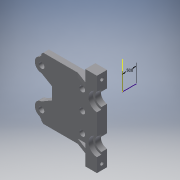
# Autodesk Inventor part: Hotend mount
Saved by Autodesk Inventor 2016 (Build 200138000, 138)
## iProperties
Created: 2016-06-02
Part Number: Hotend mount
Material: Generic
Document SubType Name: Modeling
Designer: Scott
Density: 1 g/cm^3
Appearance: Default
Author: Scott
Autodesk Inventor part; units mm, degrees
ref_plane "YZ Plane" through (0, 0, 0) normal (1, 0, 0) x (0, 1, 0)
ref_plane "XZ Plane" through (0, 0, 0) normal (0, 1, 0) x (-1, 0, 0)
sketch "Sketch1" plane through (0, 0, 0) normal (0, 0, 1) x (1, 0, 0)
  line L0 (-13.6843, -5.4848) -> (-23.1843, -10.9697) projected
  line L1 (-23.1843, -10.9697) -> (-32.6843, -5.4848) projected
  line L2 (-32.6843, -5.4848) -> (-32.6843, 5.4848) projected
  line L3 (-32.6843, 5.4848) -> (-23.1843, 10.9697) projected
  line L4 (-23.1843, 10.9697) -> (-13.6843, 5.4848) projected
  line L5 (-13.6843, 5.4848) -> (-13.6843, -5.4848) projected
  circle A0 centre (13.3507, 17.0193) radius 2.54 projected
  circle A1 centre (13.3507, -17.4028) radius 2.54 projected
  circle A2 centre (13.3507, 0) radius 2.54 projected
  circle A3 centre (-23.0489, 17.0193) radius 2.54 projected
  circle A4 centre (-23.2, -17.4028) radius 2.54 projected
  line L6 (-54.6393, -27.54) -> (18.4307, -27.54) projected
  line L7 (18.4307, -27.54) -> (18.4307, 27.54) projected
  line L8 (-54.6393, 27.54) -> (18.4307, 27.54) projected
  line L9 (-54.6393, -27.54) -> (-54.6393, 27.54) projected
  arc A5 (-23.1843, 23.0689) -> (-23.1843, 10.9697) centre (-23.0489, 17.0193) ccw
  line L10 (-23.1843, 10.9697) -> (-13.6843, 5.4848)
  line L11 (-13.6843, 5.4848) -> (-13.6843, -5.4848)
  line L12 (-13.6843, -5.4848) -> (-23.1843, -10.9697)
  line L13 (-23.1843, -23.6032) -> (-23.1843, -27.54)
  line L14 (-23.1843, 23.0689) -> (-23.1843, 27.54)
  line L15 (-23.1843, -27.54) -> (18.4307, -27.54)
  line L16 (18.4307, -27.54) -> (18.4307, 27.54)
  line L17 (18.4307, 27.54) -> (-23.1843, 27.54)
  arc A6 (-23.1843, -10.9697) -> (-23.1843, -23.6032) centre (-22.7708, -17.2864) ccw
  point P0 (0, 0)
  constraints: 16 end point, 5 collinear, 4 point on circle, 4 point on line, 2 centre point, 1 coincident, 1 horizontal, 1 perpendicular
extrude "Extrusion1" add sketch "Sketch1" along normal blind 5.08 contours L5 L4 A5 L14 L8 L7 L6 L13 A6 L0
chamfer "Chamfer1" distance 1.5875 angle 45 4 edges at (-23.1843, -27.54, 2.54) (-23.1843, 27.54, 2.54) (-23.1843, 23.0689, 2.54) (-23.1843, -23.6032, 2.54)
sketch "Sketch2" plane through (18.4307, -27.54, 0) normal (1, 0, 0) x (0, 0, -1)
  line L0 (25.4, 55.08) -> (25.4, 29.5535) projected
  line L1 (25.4, 29.5535) -> (38.1, 29.5535)
  point P0 (0, 27.54)
  dimension "d5" = 12.7
  constraints: 2 end point, 1 horizontal
  measures "d5" distance of L0.end L1.end
sketch "Sketch3" plane through (0, 0, 5.08) normal (0, 0, 1) x (1, 0, 0)
  line L0 (-23.1843, 25.9525) -> (-21.5968, 27.54) projected
  line L1 (-23.1843, 25.9525) -> (-23.1843, 24.6564) projected
  line L2 (-24.753, 22.8255) -> (-23.1843, 24.6564) projected
  arc A0 (-24.753, 22.8255) -> (-23.1843, 10.9697) centre (-23.0489, 17.0193) ccw projected
  line L3 (-23.1843, 10.9697) -> (-13.6843, 5.4848) projected
  line L4 (-13.6843, 5.4848) -> (-13.6843, -5.4848) projected
  line L5 (-13.6843, -5.4848) -> (-23.1843, -10.9697) projected
  arc A1 (-23.1843, -10.9697) -> (-24.7429, -23.3017) centre (-22.7708, -17.2864) ccw projected
  line L6 (-23.1843, -25.1907) -> (-24.7429, -23.3017) projected
  line L7 (-23.1843, -25.1907) -> (-23.1843, -25.9525) projected
  line L8 (-21.5968, -27.54) -> (-23.1843, -25.9525) projected
  line L9 (-21.5968, -27.54) -> (18.4307, -27.54) projected
  line L10 (18.4307, -27.54) -> (18.4307, 27.54) projected
  line L11 (18.4307, 27.54) -> (-21.5968, 27.54) projected
  circle A2 centre (-23.2, -17.4028) radius 2.54 projected
  circle A3 centre (-23.0489, 17.0193) radius 2.54 projected
  circle A4 centre (13.3507, 0) radius 2.54 projected
  circle A5 centre (13.3507, -17.4028) radius 2.54 projected
  circle A6 centre (13.3507, 17.0193) radius 2.54 projected
  line L12 (18.4307, -17.4028) -> (24.9307, -17.4028)
  line L13 (24.9307, -17.4028) -> (30.9307, -17.4028)
  arc A7 (30.9307, -11.4028) -> (30.9307, -23.4028) centre (30.9307, -17.4028) ccw
  line L14 (30.9307, -23.4028) -> (30.9307, -27.54)
  line L15 (30.9307, -27.54) -> (18.4307, -27.54)
  line L16 (18.4307, 0) -> (20.9229, 0)
  line L17 (18.4307, 17.4028) -> (24.9307, 17.4028)
  line L18 (24.9307, 17.4028) -> (30.9307, 17.4028)
  arc A8 (30.9307, 23.4028) -> (30.9307, 11.4028) centre (30.9307, 17.4028) ccw
  line L19 (30.9307, 23.4028) -> (30.9307, 27.54)
  line L20 (30.9307, 27.54) -> (18.4307, 27.54)
  line L21 (30.9307, -11.4028) -> (30.9307, 11.4028)
  point P0 (0, 0)
  dimension "d6" = 6.5
  dimension "d7" = 6
  dimension "d8" = 6
  constraints: 20 end point, 7 symmetric about line, 5 point on circle, 3 point on line, 2 centre point, 2 coincident, 2 perpendicular, 2 vertical, 1 horizontal, 1 midpoint, 1 other
  measures "d6" distance of L12.start L12.end
  measures "d7" distance of L12.end L13.end
  measures "d8" radius of A7
ref_plane "Work Plane1" through (-54.6393, -27.54, 0) normal (0, 0, 1) x (1, 0, 0)
extrude "Extrusion2" add sketch "Sketch3" against normal up to surface (5.08 mm away) contours L20 L19 A8 L17 L10 | L17 A8 L21 A7 L12 L10 | L12 A7 L14 L15 L10
sketch "Sketch4" plane through (0, 0, 5.08) normal (0, 0, 1) x (1, 0, 0)
  line L0 (-23.1843, 25.9525) -> (-21.5968, 27.54) projected
  line L1 (-23.1843, 25.9525) -> (-23.1843, 24.6564) projected
  line L2 (-24.753, 22.8255) -> (-23.1843, 24.6564) projected
  arc A0 (-24.753, 22.8255) -> (-23.1843, 10.9697) centre (-23.0489, 17.0193) ccw projected
  line L3 (-23.1843, 10.9697) -> (-13.6843, 5.4848) projected
  line L4 (-13.6843, 5.4848) -> (-13.6843, -5.4848) projected
  line L5 (-13.6843, -5.4848) -> (-23.1843, -10.9697) projected
  arc A1 (-23.1843, -10.9697) -> (-24.7429, -23.3017) centre (-22.7708, -17.2864) ccw projected
  line L6 (-23.1843, -25.1907) -> (-24.7429, -23.3017) projected
  line L7 (-23.1843, -25.1907) -> (-23.1843, -25.9525) projected
  line L8 (-21.5968, -27.54) -> (-23.1843, -25.9525) projected
  line L9 (-21.5968, -27.54) -> (30.9307, -27.54) projected
  line L10 (30.9307, -27.54) -> (30.9307, -23.4028) projected
  arc A2 (30.9307, -11.4028) -> (30.9307, -23.4028) centre (30.9307, -17.4028) ccw projected
  line L11 (30.9307, -11.4028) -> (30.9307, 11.4028) projected
  arc A3 (30.9307, 23.4028) -> (30.9307, 11.4028) centre (30.9307, 17.4028) ccw projected
  line L12 (30.9307, 23.4028) -> (30.9307, 27.54) projected
  line L13 (30.9307, 27.54) -> (-21.5968, 27.54) projected
  circle A4 centre (-23.2, -17.4028) radius 2.54 projected
  circle A5 centre (-23.0489, 17.0193) radius 2.54 projected
  circle A6 centre (13.3507, 0) radius 2.54 projected
  circle A7 centre (13.3507, -17.4028) radius 2.54 projected
  circle A8 centre (13.3507, 17.0193) radius 2.54 projected
  line L14 (30.9307, -23.4028) -> (30.9307, -27.54) projected
  arc A9 (30.9307, -9.4028) -> (30.9307, -25.4028) centre (30.9307, -17.4028) ccw
  arc A10 (30.9307, 23.4028) -> (30.9307, 11.4028) centre (30.9307, 17.4028) ccw projected
  line L15 (30.9307, -11.4028) -> (30.9307, 11.4028) projected
  arc A11 (30.9307, 25.4028) -> (30.9307, 9.4028) centre (30.9307, 17.4028) ccw
  line L16 (-21.5968, -27.54) -> (30.9307, -27.54) projected
  line L17 (20.0107, -27.54) -> (20.0107, 27.54)
  line L18 (30.9307, 27.54) -> (-21.5968, 27.54) projected
  line L19 (20.0107, -26.7462) -> (20.0107, -27.54)
  line L20 (-21.5968, -27.54) -> (30.9307, -27.54) projected
  line L21 (20.0107, -27.54) -> (30.9307, -27.54)
  line L22 (30.9307, -27.54) -> (30.9307, -23.4028) projected
  line L23 (30.9307, -25.4028) -> (30.9307, -27.54)
  line L24 (30.9307, -9.4028) -> (30.9307, 9.4028)
  line L25 (20.0107, 27.54) -> (30.9307, 27.54)
  line L26 (30.9307, 27.54) -> (30.9307, 25.4028)
  line L27 (30.9307, 23.4028) -> (30.9307, 27.54) projected
  point P0 (0, 0)
  dimension "d11" = 8
  dimension "d12" = 8
  constraints: 14 end point, 5 point on line, 4 collinear, 4 point on circle, 2 centre point, 2 coincident, 2 perpendicular, 1 vertical
  measures "d11" radius of A9
  measures "d12" radius of A11
extrude "Extrusion3" add sketch "Sketch4" along normal blind 4 contours L13 L12 A11 L11 A9 L10 L9 L17
sketch "Sketch5" plane through (-21.5968, -27.54, 0) normal (0, -1, 0) x (1, 0, 0)
  point P0 (21.5968, 0)
sketch "Sketch6" plane through (-21.5968, -27.54, 0) normal (0, -1, 0) x (1, 0, 0)
  line L0 (0, 0) -> (0, 5.08) projected
  line L1 (0, 0) -> (52.5275, 0) projected
  line L2 (52.5275, 0) -> (52.5275, 9.08) projected
  line L3 (41.6075, 9.08) -> (52.5275, 9.08) projected
  line L4 (41.6075, 5.08) -> (41.6075, 9.08) projected
  line L5 (0, 5.08) -> (41.6075, 5.08) projected
  line L6 (41.6075, 5.08) -> (41.6075, 9.08) projected
  line L7 (41.6075, 9.08) -> (30.9206, 5.08)
  line L8 (0, 5.08) -> (41.6075, 5.08) projected
  point P0 (21.5968, 0)
  constraints: 2 end point, 1 point on line
extrude "Extrusion4" add sketch "Sketch6" against normal blind 4 contours L7 L4 L5
sketch "Sketch7" plane through (-21.5968, 27.54, 5.08) normal (0, 1, 0) x (1, 0, 0)
  line L0 (41.6075, 0) -> (41.6075, -4) projected
  line L1 (30.9206, 0) -> (41.6075, 0) projected
  line L2 (30.9206, 0) -> (41.6075, -4) projected
  point P0 (21.5968, 5.08)
extrude "Extrusion5" add sketch "Sketch7" against normal blind 4
sketch "Sketch8" plane through (0, 0, 9.08) normal (0, 0, 1) x (1, 0, 0)
  line L0 (30.9307, -27.54) -> (30.9307, -25.4028) projected
  arc A0 (30.9307, -9.4028) -> (30.9307, -25.4028) centre (30.9307, -17.4028) ccw projected
  line L1 (30.9307, -9.4028) -> (30.9307, 9.4028) projected
  arc A1 (30.9307, 25.4028) -> (30.9307, 9.4028) centre (30.9307, 17.4028) ccw projected
  line L2 (30.9307, 25.4028) -> (30.9307, 27.54) projected
  line L3 (30.9307, 27.54) -> (20.0107, 27.54) projected
  line L4 (20.0107, 27.54) -> (20.0107, 23.54) projected
  line L5 (20.0107, 23.54) -> (20.0107, -23.54) projected
  line L6 (20.0107, -23.54) -> (20.0107, -27.54) projected
  line L7 (20.0107, -27.54) -> (30.9307, -27.54) projected
  line L8 (20.0107, 27.54) -> (30.9307, 27.54)
  line L9 (30.9307, 27.54) -> (30.9307, 37.7)
  line L10 (30.9307, 37.7) -> (20.0107, 37.7)
  line L11 (20.0107, 37.7) -> (20.0107, 27.54)
  line L12 (20.0107, -27.54) -> (30.9307, -27.54) projected
  line L13 (20.0107, -27.54) -> (30.9307, -27.54)
  line L14 (30.9307, -27.54) -> (30.9307, -37.7)
  line L15 (30.9307, -37.7) -> (20.0107, -37.7)
  line L16 (20.0107, -37.7) -> (20.0107, -27.54)
  point P0 (0, 0)
  dimension "d19" = 10.16
  dimension "d20" = 10.16
  constraints: 16 end point, 4 parallel, 2 horizontal, 2 perpendicular, 1 point on line
  measures "d19" distance of L9.end L8.end
  measures "d20" distance of L13.end L14.end
extrude "Extrusion6" add sketch "Sketch8" against normal up to surface (9.08 mm away) contours L14 L15 L16 L7 | L11 L10 L9 L3
sketch "Sketch9" plane through (30.9307, -23.4028, 5.08) normal (1, 0, 0) x (0, 0, -1)
  line L0 (5.08, 50.9428) -> (5.08, 61.1028) projected
  line L1 (-4, 50.9428) -> (5.08, 50.9428) projected
  line L2 (-4, 61.1028) -> (-4, 50.9428) projected
  line L3 (-4, 61.1028) -> (5.08, 61.1028) projected
  line L4 (5.08, -14.2972) -> (5.08, -4.1372) projected
  line L5 (-4, -14.2972) -> (5.08, -14.2972) projected
  line L6 (-4, -4.1372) -> (-4, -14.2972) projected
  line L7 (5.08, -4.1372) -> (-4, -4.1372) projected
  circle A0 centre (0.54, -9.2172) radius 1.5
  circle A1 centre (0.54, 56.0228) radius 1.5
  point P0 (5.08, 23.4028)
  dimension "d23" = 3
  dimension "d24" = 3
  constraints: 2 centre point
  measures "d23" diameter of A0
  measures "d24" diameter of A1
extrude "Extrusion7" cut sketch "Sketch9" against normal blind 18.2875 contours A0 | A1
sketch "Sketch10" plane through (30.9307, -11.4028, 0) normal (1, 0, 0) x (0, 0, -1)
  line L0 (-12.4469, -33.6461) -> (5.8759, -33.6461)
  line L1 (5.8759, -33.6461) -> (5.8759, 55.3145)
  line L2 (5.8759, 55.3145) -> (-12.4469, 55.3145)
  line L3 (-12.4469, 55.3145) -> (-12.4469, -33.6461)
  point P0 (0, 11.4028)
  constraints: 8 end point, 2 parallel, 1 horizontal, 1 perpendicular
extrude "Extrusion8" cut sketch "Sketch10" against normal blind 0.5
body "Solid1"
